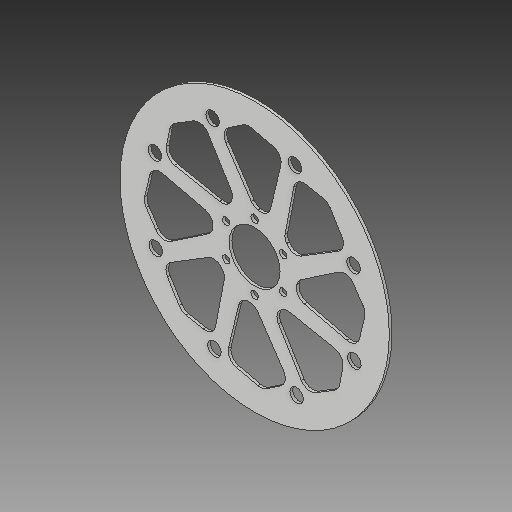
# Autodesk Inventor part: DiskBrake180
Saved by Autodesk Inventor 2019.2 (Build 232265000, 265)
## iProperties
Created: 2018-01-09
Part Number: DiskBrake180
Material: Generic
Document SubType Name: Modeling
Designer: eroldan
Density: 1 g/cm^3
Appearance: Default
Author: eroldan
Autodesk Inventor part; units mm, degrees
ref_plane "YZ Plane" through (0, 0, 0) normal (1, 0, 0) x (0, 1, 0)
ref_plane "XZ Plane" through (0, 0, 0) normal (0, 1, 0) x (-1, 0, 0)
ref_plane "XY Plane" through (0, 0, 0) normal (0, 0, 1) x (1, 0, 0)
sketch "Sketch1" plane through (0, 0, 0) normal (0, 0, 1) x (1, 0, 0)
  circle A0 centre (0, 0) radius 90
  circle A1 centre (0, 0) radius 17
  point P0 (0, 22)
  dimension "d0" = 180
  dimension "d1" = 34
  dimension "d4" = 22
  constraints: 2 centre point, 2 coincident
  measures "d0" diameter of A0
  measures "d1" diameter of A1
  measures "d4" distance of point (0, 0) point (0, 22)
extrude "Extrusion1" add sketch "Sketch1" along normal mid plane 1.8
hole "Hole1" at (0, 22, 0) direction (0, 0, -1) diameter 5 end through all both
pattern_circular "Circular Pattern1" count 6 over 360 about axis through (0, 0, -10) along (0, 0, 1) of "Hole1"
sketch "Sketch2" plane through (0, 0, 0.9) normal (0, 0, 1) x (1, 0, 0)
  line L0 (-20.7702, 19.8249) -> (-60.3067, 27.4799)
  line L1 (-60.3067, 27.4799) -> (-56.1665, 48.8634)
  line L2 (-56.1665, 48.8634) -> (-34.8846, 61.9328)
  line L3 (-34.8846, 61.9328) -> (-12.242, 25.0621)
  line L4 (-12.242, 25.0621) -> (-20.7702, 19.8249)
  circle A0 centre (-28.0858, 66.108) radius 4.5155
  point P0 (0, 0)
  constraints: 10 end point, 2 perpendicular, 1 centre point
extrude "Extrusion2" cut sketch "Sketch2" against normal blind 10
fillet "Fillet1" radius 7 5 edges at (-60.3067, 27.4799, 0) (-56.1665, 48.8634, 0) (-34.8846, 61.9328, 0) (-12.242, 25.0621, 0) (-20.7702, 19.8249, 0)
pattern_circular "Circular Pattern2" count 8 over 360 about axis through (0, 0, -10) along (0, 0, 1) of "Extrusion2", "Fillet1"
body "Solid1"
